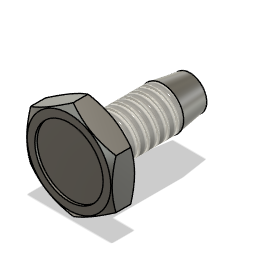
final+assembly (Autodesk Fusion 360 archive; units mm, degrees)
design "Large Indented Hex Head Tapping Screw ASME B18.6.4 4-40 UNC x 0.25 Type C Steel Grade 2 Plain"
description: Large Indented Hex Head Tapping Screw ASME B18.6.4 4-40 UNC x 0.25 Type C
part number: LIHHTSTC ASME B18.6.4 - 4-40 UNC x 0.25 Steel Grade 2 Plain
Autodesk Fusion 360 part; units mm, degrees
sketch "Sketch1" plane through (0, 0, 0) normal (0, 1, 0) x (1, 0, 0)
  line L0 (0, 6.35) -> (0, -1.3716)
  line L1 (3.2124, -0.281) -> (3.2124, -1.243)
  line L2 (3.2124, -1.243) -> (2.7257, -1.524)
  line L3 (2.7257, -1.524) -> (2.225, -1.524)
  line L4 (1.4224, 0) -> (1.4224, 6.35)
  line L5 (1.4224, 6.35) -> (0, 6.35)
  line L6 (3.2124, -0.281) -> (2.7257, 0)
  line L7 (2.7257, 0) -> (1.4224, 0)
  line L8 (2.225, -1.524) -> (2.225, -1.3716)
  line L9 (2.225, -1.3716) -> (0, -1.3716)
  line L10 (2.7257, -1.524) -> (2.7257, 0) construction
  dimension "d6" = 30
  dimension "d9" = 6.4248
  dimension "d27" = 30
  dimension "d28" = 1.524
  dimension "d50" = 2.8448
  dimension "d54" = 4.4501
  dimension "d56" = 5.4513
  dimension "d59" = 0.1524
  dimension "d60" = 6.35
  constraint vertical L0
  constraint perpendicular L0 L3
  constraint perpendicular L4 L7
  constraint coincident L0.start L5.end
  constraint coincident origin L0
  constraint coincident origin L7
  constraint perpendicular L0 L5
  constraint perpendicular L3 L8
  constraint coincident L0 L9.end
  constraint perpendicular L0 L9
  constraint coincident L0.end L9.end
  constraint perpendicular L7 L10
  measures "d6" angle of L2 L3
  measures "d27" angle of L6 L7
  measures "d28" distance of L3 L7
  measures "d59" distance of L3.end L9
  measures "d60" distance of L4.start L5
revolve "Revolve1" add sketch "Sketch1" angle 360 about axis through (0, 0, 1.75) along (0, 0, 1)
sketch "Sketch2" plane through (0, 0, 1.524) normal (0, 0, 1) x (1, 0, 0)
  circle A0 centre (0, 0) radius 2.7257
  line L0 (0, 0) -> (-2.7813, 0) construction
  line L1 (-2.7813, -1.6074) -> (-2.7813, 1.6074)
  circle A1 centre (0, 0) radius 3.2124
  circle A2 centre (0, 0) radius 2.225
  dimension "d61" = 2.7813
  constraint coincident A0.centre L0.start
  constraint horizontal L0
  constraint perpendicular L0 L1
  constraint coincident L1.end A1
  constraint coincident L1.start A1
  constraint coincident L0.end L1
  measures "d61" distance of A0.centre L1
extrude "Extrude1" cut sketch "Sketch2" against normal blind 1.524 contours L1 A1 picked at (-2.8509, 0.3915)
pattern_circular "C-Pattern1" count 6 over 360 about axis through (0, 0, 1.75) along (0, 0, 1) of "Extrude1"
thread "Thread1" "ANSI Unified Screw Threads 0.112(#4) 4-40 UNC 2A" major diameter 2.761 minor diameter 2.0676 pitch 0.635 angle 60 resizes the face on face at (1.4206, -0.0709, -4.2333)
sketch "Sketch5" plane through (0, 0, 0) normal (0, 1, 0) x (1, 0, 0)
  line L0 (0, 0) -> (0, 6.35)
  line L1 (0, 6.35) -> (-1.4508, 6.35)
  line L2 (-1.4508, 6.35) -> (-1.4508, 4.1148)
  line L3 (-1.4508, 4.1148) -> (-1.1049, 6.35)
  point P0 (0, 6.35)
  dimension "d62" = 2.2352
  dimension "d63" = 1.1049
  dimension "d64" = 1.4508
  constraint perpendicular L0 L1
  constraint perpendicular L1 L2
  constraint coincident L1 L3.end
  constraint coincident P0 L0.end
  constraint vertical L0
  measures "d62" distance of L1 L2.end
  measures "d63" distance of L0 L3.end
  measures "d64" distance of L0 L1.end
revolve "Revolve2" cut sketch "Sketch5" angle 360 about axis through (0, 0, 1.75) along (0, 0, 1)
equation "d9 = adsk_headdia"
equation "d16 = -adsk_headh"
equation "d28 = adsk_headh"
equation "adsk_nomdia = 0.112 in"
equation "adsk_nomlen = 0.25 in"
equation "adsk_headdia = 0.252945 in"
equation "adsk_waflat = 0.219 in"
equation "adsk_headh = 0.06 in"
equation "adsk_indentdia = 0.1752 in"
equation "adsk_indentdepth = 0.006 in"
equation "adsk_endpointdia = 0.087 in"
equation "d50 = adsk_nomdia"
equation "adsk_startlen = 0.088 in"
equation "d54 = adsk_indentdia"
equation "adsk_beardia = adsk_waflat * 0.98"
equation "d56 = adsk_beardia"
equation "d59 = adsk_indentdepth"
equation "d60 = adsk_nomlen"
equation "d61 = adsk_waflat / 2"
equation "d62 = adsk_startlen"
equation "d63 = adsk_endpointdia / 2"
equation "d64 = adsk_nomdia * 0.51"
